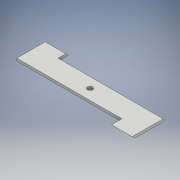
# Autodesk Inventor part: Blunt_Blade
Saved by Autodesk Inventor 2017 (Build 210142000, 142)
## iProperties
Created: 2016-10-09
Part Number: Blunt_Blade
Material: Generic
Document SubType Name: Sheet Metal
Designer: vslabsal
Density: 1 g/cm^3
Sheet Metal Rule: Default_mm
Appearance: Default
Author: vslabsal
Autodesk Inventor part; units mm, degrees
ref_plane "YZ Plane" through (0, 0, 0) normal (1, 0, 0) x (0, 1, 0)
ref_plane "XZ Plane" through (0, 0, 0) normal (0, 1, 0) x (-1, 0, 0)
ref_plane "XY Plane" through (0, 0, 0) normal (0, 0, 1) x (1, 0, 0)
sketch "Sketch1" plane through (0, 0, 0) normal (0, 0, 1) x (1, 0, 0)
  line L0 (-138.1754, -89.4085) -> (-238.1754, -89.4085)
  line L1 (-138.1754, -89.4085) -> (-138.1754, -139.4085)
  line L2 (-138.1754, -139.4085) -> (371.8246, -139.4085)
  line L3 (-240.6219, -239.4085) -> (271.8246, -239.4085)
  line L4 (271.8246, -239.4085) -> (271.8246, -289.4085)
  line L5 (371.8246, -139.4085) -> (371.8246, -289.4085)
  line L6 (271.8246, -289.4085) -> (371.8246, -289.4085)
  circle A0 centre (66.8246, -189.4085) radius 12.7
  line L7 (-238.1754, -89.4085) -> (-238.1754, -239.4085)
  dimension "d1" = 100
  dimension "d8" = 25.4
  dimension "d27" = 100
  dimension "d28" = 100
  dimension "d29" = 150
  dimension "d30" = 150
  dimension "d31" = 610
  dimension "d32" = 305
  dimension "d33" = 50
  constraints: 16 end point, 3 horizontal, 2 vertical, 1 centre point, 1 perpendicular, 1 point on line
  measures "d1" distance of L0.start L0.end
  measures "d8" diameter of A0
  measures "d27" distance between parallel lines of L5 L4
  measures "d28" distance between parallel lines of L2 L3
  measures "d29" distance between parallel lines of L3 L0
  measures "d30" distance between parallel lines of L2 L6
  measures "d31" distance between parallel lines of L7 L5
  measures "d32" distance from line of L7 A0.centre
  measures "d33" distance from line of A0.centre L3
extrude "Extrusion1" add sketch "Sketch1" along normal blind 12.7
chamfer "Chamfer1" distance 12.7 angle 45 1 edges at (-188.1754, -89.4085, 12.7)
chamfer "Chamfer2" distance 12.7 angle 45 1 edges at (321.8246, -289.4085, 0)
equation "\"BendRadius\" = Thickness"
equation "\"BendReliefWidth\" = Thickness"
equation "\"BendReliefDepth\" = 0.5 * Thickness"
equation "\"CornerReliefSize\" = 4 * Thickness"
equation "\"MinimumRemnant\" = 2 * Thickness"
equation "\"TransitionRadius\" = BendRadius"
equation "\"JacobiRadiusSize\" = BendRadius"
equation "\"GapSize\" = Thickness"
equation "\"Thickness\" = 0.5"
body "Solid1"
